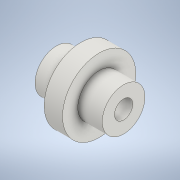
# Autodesk Inventor part: Shaft
Saved by Autodesk Inventor 2022 (Build 260153000, 153)
## iProperties
Created: 2022-03-18
Part Number: Shaft
Material: Steel
Document SubType Name: Modeling
Designer: br4ch
Density: 1 g/cm^3
Appearance: Steel
CustomPartVersion: 1
Author: br4ch
Length: 11,000 mm
Autodesk Inventor part; units mm, degrees
ref_plane "Start Plane" through (0, 0, 0) normal (1, 0, 0) x (0, 1, 0)
ref_plane "XZ Plane" through (0, 0, 0) normal (0, 1, 0) x (-1, 0, 0)
ref_plane "XY Plane" through (0, 0, 0) normal (0, 0, 1) x (1, 0, 0)
sketch "Main Sketch" plane through (0, 0, 0) normal (0, 0, 1) x (1, 0, 0)
  line L0 (0, 0) -> (11, 0)
  line L1 (0, 0) -> (0, 3.5)
  line L2 (0, 3.5) -> (4, 3.5)
  line L3 (4, 3.5) -> (4, 6)
  line L4 (7, 6) -> (7, 3.5)
  line L5 (4, 6) -> (7, 6)
  line L6 (11, 3.5) -> (11, 0)
  line L7 (7, 3.5) -> (11, 3.5)
  dimension "d3" = 7
  dimension "d4" = 12
  dimension "d5" = 7
  constraints: 16 end point, 4 horizontal, 4 vertical
  measures "d3" diameter of L2 L0
  measures "d4" diameter of L5 L0
  measures "d5" diameter of L7 L0
revolve "Revolution1" add sketch "Main Sketch" angle 360 about axis through (0, 0, 0) along (1, 0, 0)
sketch "Sketch3" plane through (0, 0, 0) normal (-1, 0, 0) x (0, 0, 1)
  circle A0 centre (0, 0) radius 1.5
  dimension "d7" = 3
  constraints: 1 centre point, 1 coincident
  measures "d7" diameter of A0
extrude "Extrusion1" cut sketch "Sketch3" against normal up to surface (11 mm away)
equation "\"Length\" = 11"
body "Solid1"
